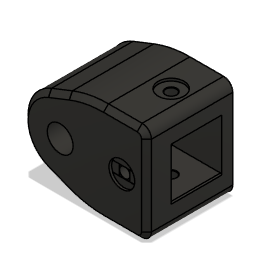
side brace upper mount v5 (Autodesk Fusion 360 design; units mm, degrees)
Autodesk Fusion 360 part; units mm, degrees
sketch "Sketch1" plane through (0, 0, 0) normal (0, 0, 1) x (1, 0, 0)
  line L0 (-40, 20.1) -> (40, 20.1)
  line L1 (40, 20.1) -> (40, -20.1)
  line L2 (40, -20.1) -> (-40, -20.1)
  line L3 (-40, -20.1) -> (-40, 20.1)
  line L4 (-40, 20.1) -> (40, -20.1) construction
  line L5 (40, 20.1) -> (-40, -20.1) construction
  line L6 (0, 20.1) -> (0, 40.1)
  line L7 (0, 40.1) -> (-50, 40.1)
  line L8 (0, -20.1) -> (0, -40.1)
  line L9 (0, -40.1) -> (-50, -40.1)
  line L10 (-40, 0) -> (-70, 0) construction
  circle A0 centre (-70, 0) radius 10.5
  circle A1 centre (-70, 0) radius 30
  line L11 (-80.978, 27.9192) -> (-50, 40.1)
  line L12 (-80.978, -27.9192) -> (-50, -40.1)
  circle A2 centre (-70, 0) radius 4.25
  dimension "d1" = 80
  dimension "d2" = 40.2
  dimension "d3" = 20
  dimension "d4" = 20
  dimension "d5" = 30
  dimension "d6" = 21
  dimension "d7" = 8.5
  dimension "d8" = 10
  dimension "d9" = 10
  constraint horizontal L0
  constraint perpendicular L0 L1
  constraint parallel L0 L2
  constraint parallel L1 L3
  constraint coincident L4 origin
  constraint coincident L5 origin
  constraint midpoint L0 L6.start
  constraint perpendicular L0 L6
  constraint perpendicular L6 L7
  constraint midpoint L2 L8.start
  constraint perpendicular L2 L8
  constraint perpendicular L8 L9
  constraint midpoint L3 L10.start
  constraint perpendicular L3 L10
  constraint coincident L10.end A0.centre
  constraint concentric A0 A1
  constraint coincident L10.start A1
  constraint coincident A1 L11.start
  constraint tangent A1 L11
  constraint coincident A1 L12.start
  constraint tangent A1 L12
  constraint concentric A0 A2
  constraint coincident L9.end L12.end
  measures "d1" distance of L1.end L2.end
  measures "d2" distance of L0.end L1.end
  measures "d3" distance of L6.start L6.end
  measures "d4" distance of L8.start L8.end
  measures "d5" distance of L10.start L10.end
  measures "d6" diameter of A0
  measures "d7" diameter of A2
  measures "d8" horizontal distance of L2.end L9.end
  measures "d9" horizontal distance of L0.start L7.end
extrude "Extrude1" add sketch "Sketch1" along normal blind 40 contours L0 L3 L6 L7 A1 L11 | A1 | L2 L3 L8 L9 A1 L12 | A0 makes body 1
sketch "Sketch2" plane through (0, 0, 40) normal (0, 0, 1) x (1, 0, 0)
  circle A0 centre (-70, 0) radius 4.25
  arc A1 (-80.978, 27.9192) -> (-80.978, -27.9192) centre (-70, 0) ccw
  line L0 (-80.978, -27.9192) -> (-50, -40.1)
  line L1 (-50, -40.1) -> (0, -40.1)
  line L2 (0, -40.1) -> (0, -20.1)
  line L3 (0, -20.1) -> (-40, -20.1)
  line L4 (-40, -20.1) -> (-40, 20.1)
  line L5 (-40, 20.1) -> (0, 20.1)
  line L6 (0, 20.1) -> (0, 40.1)
  line L7 (0, 40.1) -> (-50, 40.1)
  line L8 (-50, 40.1) -> (-80.978, 27.9192)
  line L9 (0, 20.1) -> (0, -20.1)
  constraint coincident L5.end L6.start
  constraint coincident L2.end L3.start
extrude "Extrude2" add sketch "Sketch2" along normal blind 20 bodies 1
sketch "Sketch3" plane through (0, 0, 40) normal (0, 0, -1) x (-1, 0, 0)
  line L0 (40, 20.1) -> (0, 20.1)
  line L1 (0, 20.1) -> (0, -20.1)
  line L2 (0, -20.1) -> (40, -20.1)
  line L3 (40, -20.1) -> (40, 20.1)
  line L4 (20, 20.1) -> (20, -20.1) construction
  circle A0 centre (20, 0) radius 10.5
  circle A1 centre (20, 0) radius 4.25
  dimension "d63" = 21
  dimension "d64" = 8.5
  constraint midpoint L0 L4.start
  constraint midpoint L2 L4.end
  constraint midpoint L4 A0.centre
  constraint concentric A0 A1
  measures "d63" diameter of A0
  measures "d64" diameter of A1
extrude "Extrude16" cut sketch "Sketch3" against normal blind 38 contours A0 | A1 bodies 1
extrude "Extrude17" add sketch "Sketch3" against normal blind 18 contours A0 bodies 1
sketch "Sketch11" plane through (0, 0, 58) normal (0, 0, 1) x (1, 0, 0)
  circle A0 centre (-20, 0) radius 4.25
  circle A1 centre (-20, 0) radius 10.5
  line L0 (-29.6014, 4.25) -> (-10.3986, 4.25)
  line L1 (-10.3986, -4.25) -> (-29.6014, -4.25)
  line L2 (-15.75, 4.25) -> (-15.75, -4.25)
  line L3 (-24.25, 4.25) -> (-24.25, -4.25)
  constraint coincident A1 L0.start
  constraint coincident A1 L0.end
  constraint horizontal L0
  constraint coincident A1 L1.start
  constraint coincident A1 L1.end
  constraint parallel L0 L1
  constraint tangent A0 L1
  constraint tangent A0 L0
  constraint coincident L0 L2.start
  constraint coincident L1 L2.end
  constraint perpendicular L1 L2
  constraint coincident L0 L3.start
  constraint coincident L1 L3.end
  constraint perpendicular L1 L3
  constraint tangent A0 L3
  constraint tangent A0 L2
extrude "Extrude18" cut sketch "Sketch11" against normal blind 0.2 contours A0 L1 L2 | A0 L0 L2 | A1 L0 L1 L2 | A0 L0 L3 | A0 L1 L3 | A1 L0 L1 L3 bodies 1
extrude "Extrude19" cut sketch "Sketch11" against normal blind 0.4 contours A0 L1 L2 | A0 L0 L2 | A0 L0 L3 | A0 L1 L3 bodies 1
sketch "Sketch5" plane through (0, 0, 60) normal (0, 0, 1) x (1, 0, 0)
  circle A0 centre (-70, 0) radius 4.25
  line L0 (0, 40.1) -> (-50, 40.1)
  line L1 (-50, 40.1) -> (-80.978, 27.9192)
  arc A1 (-80.978, 27.9192) -> (-80.978, -27.9192) centre (-70, 0) ccw
  line L2 (-80.978, -27.9192) -> (-50, -40.1)
  line L3 (-50, -40.1) -> (0, -40.1)
  line L4 (0, -40.1) -> (0, 40.1)
  circle A2 centre (-70, 0) radius 10.5
  circle A3 centre (-20, 0) radius 10.5
  dimension "d24" = 21
  constraint concentric A0 A2
  measures "d24" diameter of A2
extrude "Extrude5" cut sketch "Sketch5" against normal blind 22 contours A2 bodies 1
sketch "Sketch8" plane through (0, 20.1, 0) normal (0, -1, 0) x (1, 0, 0)
  line L0 (-40, 0) -> (0, 0)
  line L1 (0, 0) -> (0, 40)
  line L2 (0, 40) -> (-40, 40)
  line L3 (-40, 40) -> (-40, 0)
  line L4 (-40, 40) -> (0, 0) construction
  circle A0 centre (-20, 20) radius 4.25
  circle A1 centre (-20, 20) radius 10.5
  dimension "d42" = 8.5
  dimension "d43" = 21
  constraint coincident L2.end L3.start
  constraint coincident L0.end L1.start
  constraint midpoint L4 A0.centre
  constraint concentric A0 A1
  measures "d42" diameter of A0
  measures "d43" diameter of A1
extrude "Extrude9" cut sketch "Sketch8" along normal blind -43 and the other way blind -83 contours A0 | A1 bodies 1
extrude "Extrude10" add sketch "Sketch8" against normal blind 18 contours A1 bodies 1
extrude "Extrude11" add sketch "Sketch8" along normal blind 18 from surface at 40.2 contours A1 bodies 1
sketch "Sketch10" plane through (0, 0, 38) normal (0, 0, 1) x (1, 0, 0)
  circle A0 centre (-70, 0) radius 4.25
  circle A1 centre (-70, 0) radius 10.5
  line L0 (-74.25, 9.6014) -> (-74.25, -9.6014)
  line L1 (-65.75, 9.6014) -> (-65.75, -9.6014)
  line L2 (-74.25, 4.25) -> (-65.75, 4.25)
  line L3 (-65.75, -4.25) -> (-74.25, -4.25)
  constraint coincident A1 L0.start
  constraint coincident A1 L0.end
  constraint vertical L0
  constraint coincident A1 L1.start
  constraint coincident A1 L1.end
  constraint parallel L0 L1
  constraint coincident L0 L2.start
  constraint coincident L1 L2.end
  constraint perpendicular L1 L2
  constraint coincident L1 L3.start
  constraint coincident L0 L3.end
  constraint perpendicular L0 L3
  constraint tangent A0 L3
  constraint tangent A0 L1
  constraint tangent A0 L2
  constraint tangent A0 L0
extrude "Extrude14" cut sketch "Sketch10" against normal blind 0.2 contours A0 L1 L3 | A0 L1 L2 | A0 L0 L2 | A1 L0 L1 L2 | A0 L0 L3 | A1 L0 L1 L3 bodies 1
extrude "Extrude15" cut sketch "Sketch10" against normal blind 0.4 contours A0 L1 L3 | A0 L1 L2 | A0 L0 L2 | A0 L0 L3 bodies 1
extrude "Extrude20" add 1 faces at (-48.5833, 0, 0) along direction (0, 0, -1) blind 10 on bodies 1 bodies 1
sketch "Sketch12" plane through (-40, 0, 0) normal (1, 0, 0) x (0, 0, -1)
  line L0 (10, 20.1) -> (-40, 20.1)
  line L1 (-40, 20.1) -> (-40, -20.1)
  line L2 (-40, -20.1) -> (10, -20.1)
  line L3 (10, -20.1) -> (10, 20.1)
  line L4 (1, 20.1) -> (1, -20.1)
  dimension "d85" = 41
  constraint coincident L0 L4.start
  constraint coincident L2 L4.end
  constraint perpendicular L2 L4
  measures "d85" distance of L1 L4
extrude "Extrude21" add sketch "Sketch12" along normal blind 40 contours L0 L2 L3 L4 bodies 1
fillet "Fillet2" radius 80 2 edges at (-50, 40.1, 30) (-50, -40.1, 30) on bodies 1
fillet "Fillet2" radius 7.5 2 edges at (0, 40.1, 30) (0, -40.1, 30) on bodies 1
chamfer "Chamfer1" distance 4 distance2 4 10 edges at (-49.7348, 38.7006, 60) (-21.1684, 40.1, 60) (-2.1967, 37.9033, 60) (0, 0, 60) (-2.1967, -37.9033, 60) (-21.1684, -40.1, 60) (-49.7348, -38.7006, 60) (-72.5448, -31.2352, 60) (-100, 0, 60) (-72.5448, 31.2352, 60) measured on face at (-51.3673, 38.3735, 36.6667) measured on face at (-44.9337, 17.1022, 60) measured on face at (-7.1431, 40.0915, 36.6667) measured on face at (-44.9337, 17.1022, 60) measured on face at (-7.1431, -40.0915, 13.3333) measured on face at (-44.9337, 17.1022, 60) measured on face at (-38.1659, -40.0307, 13.3333) measured on face at (-44.9337, 17.1022, 60) measured on face at (-44.9337, 17.1022, 60) measured on face at (-44.9337, 17.1022, 60) on bodies 1
chamfer "Chamfer1" distance 0.4 distance2 0.4 2 edges at (-16.0376, 1.5369, 40) (-73.9624, -1.5369, -10) 2 faces at (-15.7553, -32.1, 19.7882) (-15.7553, 32.1, 19.7882) measured on face at (-20.1059, -14.8127, 40) measured on face at (-21.9167, 0, -10) on bodies 1
fillet "Fillet3" radius 1 2 edges at (0, -20.1, 20) (0, 20.1, 20) on bodies 1
copy_body "Body->Comp1" bodies 1 removing the originals makes body 2 in component "side brace upper mount"
component "side brace upper mount" placed x (1, 0, 0) y (0, 1, 0) z (0, 0, 1) at (0, 0, 0)
named bodies: "side brace upper mount"
